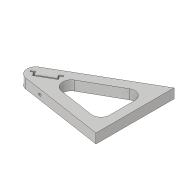
# Autodesk Inventor part: Din_Rail_0.45mm_Clearance
Saved by Autodesk Inventor 2017 SP1 (Build 210196100, 196)
## iProperties
Created: 2016-06-09
Part Number: Din_Rail_0.45mm_Clearance
Material: Generic
Document SubType Name: Modeling
Designer: Tom
Density: 1 g/cm^3
Appearance: Default
Author: Tom
Autodesk Inventor part; units mm, degrees
ref_plane "YZ Plane" through (0, 0, 0) normal (1, 0, 0) x (0, 1, 0)
ref_plane "XZ Plane" through (0, 0, 0) normal (0, 1, 0) x (-1, 0, 0)
ref_plane "XY Plane" through (0, 0, 0) normal (0, 0, 1) x (1, 0, 0)
sketch "Sketch1" plane through (0, 0, 0) normal (0, 1, 0) x (-1, 0, 0)
  line L0 (0, 0) -> (0, -114.3)
  line L1 (0, -114.3) -> (125.3564, -41.9254)
  line L2 (0, -114.3) -> (144.7491, -114.3) construction
  line L3 (120.9141, -18.371) -> (0, 0)
  arc A0 (125.3564, -41.9254) -> (120.9141, -18.371) centre (119.0064, -30.9269) ccw
  line L4 (12.7, -32.7621) -> (12.7, -69.4305)
  line L5 (0, -114.3) -> (0, -98.425)
  line L6 (31.6623, -80.4792) -> (82.681, -51.5623)
  line L7 (78.3264, -27.9577) -> (27.3077, -20.2062)
  arc A1 (82.681, -51.5623) -> (78.3264, -27.9577) centre (76.4188, -40.5136) ccw
  arc A2 (12.7, -69.4305) -> (31.6623, -80.4792) centre (25.4, -69.4305) ccw
  arc A3 (27.3077, -20.2062) -> (12.7, -32.7621) centre (25.4, -32.7621) ccw
  line L8 (126.7827, -31.0259) -> (121.8464, -33.8759)
  line L9 (121.8464, -33.8759) -> (118.7464, -28.5065)
  line L10 (126.7827, -31.0259) -> (125.9327, -29.5536)
  line L11 (125.9327, -29.5536) -> (122.4686, -31.5536)
  line L12 (122.4686, -31.5536) -> (119.4686, -26.3575)
  line L13 (118.7464, -28.5065) -> (108.1376, -34.6315)
  line L14 (119.4686, -26.3575) -> (107.3876, -33.3325)
  line L15 (95.6924, -48.9759) -> (100.6288, -46.1259)
  line L16 (100.6288, -46.1259) -> (97.5288, -40.7565)
  line L17 (95.6924, -48.9759) -> (94.8424, -47.5036)
  line L18 (94.8424, -47.5036) -> (98.3065, -45.5036)
  line L19 (98.3065, -45.5036) -> (95.3065, -40.3075)
  line L20 (97.5288, -40.7565) -> (108.1376, -34.6315)
  line L21 (95.3065, -40.3075) -> (107.3876, -33.3325)
  point P0 (156.7289, -23.8125)
  dimension "d0" = 114.3
  dimension "d2" = 30
  dimension "d3" = 12.7
  dimension "d5" = 15.875
  dimension "d8" = 12.7
  dimension "d9" = 12.7
  dimension "d34" = 5.7
  dimension "d36" = 6.2
  dimension "d37" = 1.7
  dimension "d38" = 4
  dimension "d39" = 6
  dimension "d41" = 12.25
  dimension "d42" = 13.95
  dimension "d45" = 1.7
  dimension "d46" = 12.25
  dimension "d47" = 13.95
  dimension "d48" = 1.7
  dimension "d49" = 6.2
  dimension "d50" = 5.7
  dimension "d59" = 24.5
  constraints: 44 end point, 8 point on circle, 8 tangent, 4 centre point, 2 perpendicular, 2 point on line, 1 equal length, 1 equal radius, 1 horizontal, 1 parallel, 1 vertical
  measures "d0" distance of L0.start L0.end
  measures "d2" angle of L2 L1
  measures "d3" radius of A0
  measures "d5" distance of L0.end L5.end
  measures "d8" radius of A1
  measures "d9" radius of A2
  measures "d34" distance of L8.start L8.end
  measures "d36" distance of L8.end L9.end
  measures "d37" distance of L8.start L10.end
  measures "d38" distance of L10.end L11.end
  measures "d39" distance of L11.end L12.end
  measures "d41" distance of L9.end L13.end
  measures "d42" distance of L12.end L14.end
  measures "d45" distance between parallel lines of L9 L12
  measures "d46" distance from line of L16 L13.end
  measures "d47" distance from line of L19 L14.end
  measures "d48" distance between parallel lines of L15 L18
  measures "d49" distance between parallel lines of L15 L20
  measures "d50" distance between parallel lines of L17 L16
  measures "d59" distance between parallel lines of L16 L9
extrude "Extrusion2" add sketch "Sketch1" along normal blind 14
sketch "Sketch3" plane through (-97.5288, 0, -40.7565) normal (0.5, 0, 0.866) x (0.866, 0, -0.5)
  line L0 (-13.75, 7) -> (-10.75, 7) construction
  line L1 (-13.75, 2) -> (-10.75, 2)
  line L2 (-10.75, 12) -> (-13.75, 12)
  arc A0 (-13.75, 12) -> (-13.75, 2) centre (-13.75, 7) ccw
  arc A1 (-10.75, 2) -> (-10.75, 12) centre (-10.75, 7) ccw
  line L3 (0, 0) -> (-24.5, 0) projected
  line L4 (-24.5, 0) -> (-24.5, 14) projected
  point P0 (64.0841, 0)
  point P1 (-12.25, 7)
  dimension "d55" = 10
  dimension "d56" = 7
  dimension "d57" = 3
  dimension "d58" = 12.25
  constraints: 8 end point, 4 point on circle, 4 tangent, 2 centre point, 1 horizontal, 1 midpoint, 1 parallel
  measures "d55" diameter of A1
  measures "d56" distance from line of L3 point (-12.25, 7)
  measures "d57" distance of L0.end L0.start
  measures "d58" distance from line of L4 point (-12.25, 7)
extrude "Extrusion3" cut sketch "Sketch3" against normal up to next
sketch "Sketch4" plane through (-125.3564, 0, -41.9254) normal (-0.5, 0, -0.866) x (-0.866, 0, 0.5)
  arc A0 (-9.765, 2) -> (-9.765, 12) centre (-9.765, 7) ccw projected
  arc A1 (-12.765, 12) -> (-12.765, 2) centre (-12.765, 7) ccw projected
  line L0 (-9.765, 12) -> (-12.765, 12)
  line L1 (-9.765, 2) -> (-12.765, 2) projected
  line L2 (-9.765, 12) -> (-12.765, 2)
  line L3 (-9.765, 2) -> (-12.765, 12)
  circle A2 centre (-11.265, 7) radius 1.65
  point P0 (-87.5991, 0)
  dimension "d62" = 3.3
  constraints: 6 end point, 1 centre point, 1 midpoint
  measures "d62" diameter of A2
extrude "Extrusion4" cut sketch "Sketch4" against normal up to next contours A2 L2 L3 | L3 L2 A2 | L2 L3 A2 | A2 L3 L2
body "Solid2"
